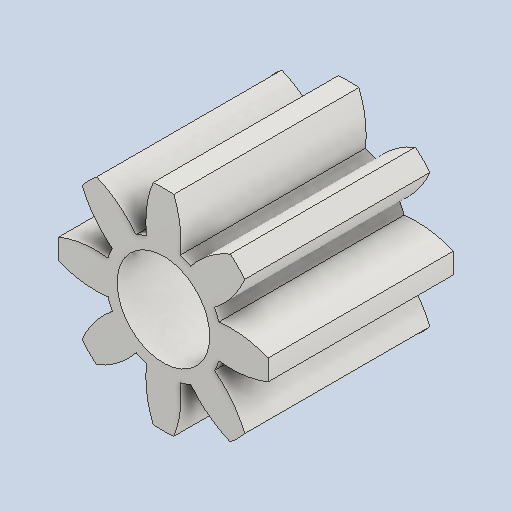
# Autodesk Inventor part: Spur Gear1
Saved by Autodesk Inventor 2022.3 (Build 263350000, 350)
## iProperties
CustomPartVersion: 1
Created: 2023-01-16
Part Number: Spur Gear1
Material: Steel
Document SubType Name: Modeling
Designer: komputer
Categories: <?xml version="1.0" encoding="UTF-16"?> <MemberInstance><Categories><FamilyTemplate><FamilyTemplateParameter ValueType="xs:double" Id="1" ObjectReferenceKey="da_z" ObjectType="kUserParameterObject"/><FamilyTemplateParameter ValueType="xs:double" Id="2" ObjectReferenceKey="da_b" ObjectType="kUserParameterObject"/><FamilyTemplateParameter ValueType="xs:double" Id="3" ObjectReferenceKey="da_beta" ObjectType="kUserParameterObject"/><FamilyTemplateParameter ValueType="xs:double" Id="4" ObjectReferenceKey="da_da" ObjectType="kUserParameterObject"/><FamilyTemplateParameter ValueType="xs:double" Id="5" ObjectReferenceKey="da_aw" ObjectType="kUserParameterObject"/><FamilyTemplateParameter ValueType="xs:string" Id="6" ObjectReferenceKey="EAIAABAAAACIAQAAAAAAAIAAAAAAAAAA" ObjectType="83910656" SubObjectId="SurfaceGeometry"/></FamilyTemplate><ParamToTemplateMap><ParamToTemplate CategoryParameter="//CategoryParameter[@InternalName='046C89C9-8512-4d59-83FE-43B91F4F132A']" TemplateParameter="1"/><ParamToTemplate CategoryParameter="//CategoryParameter[@InternalName='2552DF32-E462-4b46-AEBF-C6C7768E72AC']" TemplateParameter="2"/><ParamToTemplate CategoryParameter="//CategoryParameter[@InternalName='C9EE641D-15FC-4fae-A226-E94C4372FDD7']" TemplateParameter="3"/><ParamToTemplate><ParamToTemplate CategoryParameter="//CategoryParameter[@InternalName='00B6519A-459B-49c7-AD84-2E56D39A5744']" ConstantValue="0.000000"/></ParamToTemplate><ParamToTemplate><ParamToTemplate CategoryParameter="//CategoryParameter[@InternalName='04B31F0E-C7A6-4894-AA32-9629BEFACF47']" ConstantValue="1.000000"/></ParamToTemplate><ParamToTemplate><ParamToTemplate CategoryParameter="//CategoryParameter[@InternalName='43CBEC2E-7847-49e7-A936-2F7889FCB2D9']" ConstantValue="0.250000"/></ParamToTemplate><ParamToTemplate><ParamToTemplate CategoryParameter="//CategoryParameter[@InternalName='B1EFC894-105D-4ebd-86BF-FA20ED196853']" ConstantValue="0.350000"/></ParamToTemplate><ParamToTemplate><ParamToTemplate CategoryParameter="//CategoryParameter[@InternalName='51175063-3D10-4879-93E8-6246FE8B403D']" ConstantValue="2060000000.000000"/></ParamToTemplate><ParamToTemplate><ParamToTemplate CategoryParameter="//CategoryParameter[@InternalName='A3A52E27-4454-46a9-B0BD-C932399B70AF']" ConstantValue="0.300000"/></ParamToTemplate><ParamToTemplate><ParamToTemplate CategoryParameter="//CategoryParameter[@InternalName='91B76062-C214-41d9-B1B9-14D2AB99603D']" ConstantValue="0.045480"/></ParamToTemplate><ParamToTemplate><ParamToTemplate CategoryParameter="//CategoryParameter[@InternalName='374E806E-8B8A-4dda-A9AA-1039D6500AD2']" ConstantValue="21.987687"/></ParamToTemplate><ParamToTemplate><ParamToTemplate CategoryParameter="//CategoryParameter[@InternalName='2D373A89-B862-43d6-8D0B-0CBF12AB9F6C']" ConstantValue="0.349066"/></ParamToTemplate><ParamToTemplate CategoryParameter="//CategoryParameter[@InternalName='37777632-D6A2-4fac-9D53-DB8ACD95C989']" TemplateParameter="4"/><ParamToTemplate CategoryParameter="//CategoryParameter[@InternalName='FD1017F1-B727-4f7e-9707-0F86F1FF9423']" TemplateParameter="5"/><ParamToTemplate><ParamToTemplate CategoryParameter="//CategoryParameter[@InternalName='9E1B4470-B2D3-4ff1-B813-535BB4CDF51A']" ConstantValue="3520000.000000"/></ParamToTemplate><ParamToTemplate><ParamToTemplate CategoryParameter="//CategoryParameter[@InternalName='F8452263-BFF6-458c-9FB1-07C4B99E95CD']" ConstantValue="11400000.000000"/></ParamToTemplate><ParamToTemplate><ParamToTemplate CategoryParameter="//CategoryParameter[@InternalName='3E3BB259-FD49-497f-8171-6EBC954A3479']" ConstantValue="2.000000"/></ParamToTemplate><ParamToTemplate CategoryParameter="//CategoryParameter[@InternalName='27C3BAF2-7550-4e4b-AE2C-0DB134B7D9B7']" TemplateParameter="6"/></ParamToTemplateMap><Category DisplayName="Gear" InternalName="DC85795E-93AB-48d5-8EEE-5A27447B64BD" Mnemonic="Gear"><CategoryParameter DisplayName="z" InternalName="046C89C9-8512-4d59-83FE-43B91F4F132A" Mnemonic="z"/><CategoryParameter DisplayName="b" InternalName="2552DF32-E462-4b46-AEBF-C6C7768E72AC" Mnemonic="b"/><CategoryParameter DisplayName="||b|" InternalName="C9EE641D-15FC-4fae-A226-E94C4372FDD7" Mnemonic="beta"/><CategoryParameter DisplayName="x" InternalName="00B6519A-459B-49c7-AD84-2E56D39A5744" Mnemonic="x"/><CategoryParameter DisplayName="a*" InternalName="04B31F0E-C7A6-4894-AA32-9629BEFACF47" Mnemonic="a"/><CategoryParameter DisplayName="c*" InternalName="43CBEC2E-7847-49e7-A936-2F7889FCB2D9" Mnemonic="c"/><CategoryParameter DisplayName="r|.f|*" InternalName="B1EFC894-105D-4ebd-86BF-FA20ED196853" Mnemonic="rf"/><CategoryParameter DisplayName="E" InternalName="51175063-3D10-4879-93E8-6246FE8B403D" Mnemonic="E"/><CategoryParameter DisplayName="||m|" InternalName="A3A52E27-4454-46a9-B0BD-C932399B70AF" Mnemonic="mi"/><Category DisplayName="SpurGear" InternalName="26C5A22E-A91E-4dfd-A3B3-23CCAFAE1764" Mnemonic="SpurGear"><CategoryParameter DisplayName="m" InternalName="91B76062-C214-41d9-B1B9-14D2AB99603D" Mnemonic="m"/><CategoryParameter DisplayName="P" InternalName="374E806E-8B8A-4dda-A9AA-1039D6500AD2" Mnemonic="PP"/><CategoryParameter DisplayName="||a|" InternalName="2D373A89-B862-43d6-8D0B-0CBF12AB9F6C" Mnemonic="alpha"/><CategoryParameter DisplayName="d|.a|" InternalName="37777632-D6A2-4fac-9D53-DB8ACD95C989" Mnemonic="da"/><CategoryParameter DisplayName="a|.w|" InternalName="FD1017F1-B727-4f7e-9707-0F86F1FF9423" Mnemonic="aw"/><CategoryParameter DisplayName="||s||.Flim|" InternalName="9E1B4470-B2D3-4ff1-B813-535BB4CDF51A" Mnemonic="sFlim"/><CategoryParameter DisplayName="||s||.Hlim|" InternalName="F8452263-BFF6-458c-9FB1-07C4B99E95CD" Mnemonic="sHlim"/><CategoryParameter DisplayName="type" InternalName="3E3BB259-FD49-497f-8171-6EBC954A3479" Mnemonic="type"/><CategoryParameter DisplayName="PitchDiameter" InternalName="27C3BAF2-7550-4e4b-AE2C-0DB134B7D9B7" Mnemonic="IDS_PITCHDIAM"/></Category></Category></Categories></MemberInstance>
Density: 1 g/cm^3
Appearance: Steel
Author: komputer
Autodesk Inventor part; units mm, degrees
sketch "Sketch1" plane through (0, 0, 0) normal (0, 0, 1) x (1, 0, 0)
  circle A0 centre (0, 0) radius 2.274
  dimension "d0" = 4.548
  constraints: 1 centre point
  measures "d0" diameter of A0
extrude "Extrusion1" add sketch "Sketch1" along normal blind 20
ref_plane "Work Plane2" through (0, 0, 10) normal (0, 0, 1) x (1, 0, 0)
sketch "Sketch2" plane through (0, 0, 0) normal (0, 0, -1) x (-1, 0, 0)
  circle A0 centre (0, 0) radius 2.274 projected
  circle A1 centre (0, 0) radius 1.8192
  dimension "d3" = 3.6384
  constraints: 1 centre point, 1 coincident
  measures "d3" diameter of A1
surface extrude "Pitch Diameter" sketch "Sketch2" against normal through all shown no curves A1
ref_plane "Work Plane8" through (0, 0, 0) normal (0.9238795, 0.3826834, 0) x (0, 0, 1)
ref_plane "Work Plane9" through (0, 0, 0) normal (1, 0, 0) x (0, 1, 0)
spur gear teeth "Spur Gear" teeth 8 pitch diameter 3.6384 tip diameter 4.548 root diameter 2.5014 face width 20 start plane through (0, 0, 0) normal (0, 0, -1) x (-1, 0, 0)
sketch "Sketch3" plane through (0, 0, 20) normal (0, 0, 1) x (1, 0, 0)
  arc A0 (-1.7578, 1.4426) -> (-1.103, 0.5896) centre (0.2047, 2.2712) ccw projected
  arc A1 (-1.103, 0.5896) -> (-1.1968, 0.3631) centre (0, 0) ccw projected
  arc A2 (-1.1968, 0.3631) -> (-2.2631, 0.2229) centre (-1.4613, -1.7508) ccw projected
  arc A3 (-2.2631, 0.2229) -> (-2.2631, -0.2229) centre (0, 0) ccw projected
  arc A4 (-2.2631, -0.2229) -> (-1.1968, -0.3631) centre (-1.4613, 1.7508) ccw projected
  arc A5 (-1.1968, -0.3631) -> (-1.103, -0.5896) centre (0, 0) ccw projected
  arc A6 (-1.103, -0.5896) -> (-1.7578, -1.4426) centre (0.2047, -2.2712) ccw projected
  arc A7 (-1.7578, -1.4426) -> (-1.4426, -1.7578) centre (0, 0) ccw projected
  arc A8 (-1.4426, -1.7578) -> (-0.5896, -1.103) centre (-2.2712, 0.2047) ccw projected
  arc A9 (-0.5896, -1.103) -> (-0.3631, -1.1968) centre (0, 0) ccw projected
  arc A10 (-0.3631, -1.1968) -> (-0.2229, -2.2631) centre (1.7508, -1.4613) ccw projected
  arc A11 (-0.2229, -2.2631) -> (0.2229, -2.2631) centre (0, 0) ccw projected
  arc A12 (0.2229, -2.2631) -> (0.3631, -1.1968) centre (-1.7508, -1.4613) ccw projected
  arc A13 (0.3631, -1.1968) -> (0.5896, -1.103) centre (0, 0) ccw projected
  arc A14 (0.5896, -1.103) -> (1.4426, -1.7578) centre (2.2712, 0.2047) ccw projected
  arc A15 (1.4426, -1.7578) -> (1.7578, -1.4426) centre (0, 0) ccw projected
  arc A16 (1.7578, -1.4426) -> (1.103, -0.5896) centre (-0.2047, -2.2712) ccw projected
  arc A17 (1.103, -0.5896) -> (1.1968, -0.3631) centre (0, 0) ccw projected
  arc A18 (1.1968, -0.3631) -> (2.2631, -0.2229) centre (1.4613, 1.7508) ccw projected
  arc A19 (2.2631, -0.2229) -> (2.2631, 0.2229) centre (0, 0) ccw projected
  arc A20 (2.2631, 0.2229) -> (1.1968, 0.3631) centre (1.4613, -1.7508) ccw projected
  arc A21 (1.1968, 0.3631) -> (1.103, 0.5896) centre (0, 0) ccw projected
  arc A22 (1.103, 0.5896) -> (1.7578, 1.4426) centre (-0.2047, 2.2712) ccw projected
  arc A23 (1.7578, 1.4426) -> (1.4426, 1.7578) centre (0, 0) ccw projected
  arc A24 (1.4426, 1.7578) -> (0.5896, 1.103) centre (2.2712, -0.2047) ccw projected
  arc A25 (0.5896, 1.103) -> (0.3631, 1.1968) centre (0, 0) ccw projected
  arc A26 (0.3631, 1.1968) -> (0.2229, 2.2631) centre (-1.7508, 1.4613) ccw projected
  arc A27 (0.2229, 2.2631) -> (-0.2229, 2.2631) centre (0, 0) ccw projected
  arc A28 (-0.2229, 2.2631) -> (-0.3631, 1.1968) centre (1.7508, 1.4613) ccw projected
  arc A29 (-0.3631, 1.1968) -> (-0.5896, 1.103) centre (0, 0) ccw projected
  arc A30 (-0.5896, 1.103) -> (-1.4426, 1.7578) centre (-2.2712, -0.2047) ccw projected
  arc A31 (-1.4426, 1.7578) -> (-1.7578, 1.4426) centre (0, 0) ccw projected
ref_plane "Work Plane11" through (-4.2612, 0.6505, 4) normal (0, 0, 1) x (0.9749279, -0.2225209, 0)
extrude "Extrusion2" cut sketch "Sketch3" against normal up to surface (16 mm away)
sketch "Sketch4" plane through (0, 0, 4) normal (0, 0, 1) x (1, 0, 0)
  arc A0 (-1.1968, 0.3631) -> (-2.2631, 0.2229) centre (-1.4613, -1.7508) ccw projected
  arc A1 (-2.2631, 0.2229) -> (-2.2631, -0.2229) centre (0, 0) ccw projected
  arc A2 (-2.2631, -0.2229) -> (-1.1968, -0.3631) centre (-1.4613, 1.7508) ccw projected
  arc A3 (-1.1968, -0.3631) -> (-1.103, -0.5896) centre (0, 0) ccw projected
  arc A4 (-1.103, -0.5896) -> (-1.7578, -1.4426) centre (0.2047, -2.2712) ccw projected
  arc A5 (-1.7578, -1.4426) -> (-1.4426, -1.7578) centre (0, 0) ccw projected
  arc A6 (-1.4426, -1.7578) -> (-0.5896, -1.103) centre (-2.2712, 0.2047) ccw projected
  arc A7 (-0.5896, -1.103) -> (-0.3631, -1.1968) centre (0, 0) ccw projected
  arc A8 (-0.3631, -1.1968) -> (-0.2229, -2.2631) centre (1.7508, -1.4613) ccw projected
  arc A9 (-0.2229, -2.2631) -> (0.2229, -2.2631) centre (0, 0) ccw projected
  arc A10 (0.2229, -2.2631) -> (0.3631, -1.1968) centre (-1.7508, -1.4613) ccw projected
  arc A11 (0.3631, -1.1968) -> (0.5896, -1.103) centre (0, 0) ccw projected
  arc A12 (0.5896, -1.103) -> (1.4426, -1.7578) centre (2.2712, 0.2047) ccw projected
  arc A13 (1.4426, -1.7578) -> (1.7578, -1.4426) centre (0, 0) ccw projected
  arc A14 (1.7578, -1.4426) -> (1.103, -0.5896) centre (-0.2047, -2.2712) ccw projected
  arc A15 (1.103, -0.5896) -> (1.1968, -0.3631) centre (0, 0) ccw projected
  arc A16 (1.1968, -0.3631) -> (2.2631, -0.2229) centre (1.4613, 1.7508) ccw projected
  arc A17 (2.2631, -0.2229) -> (2.2631, 0.2229) centre (0, 0) ccw projected
  arc A18 (2.2631, 0.2229) -> (1.1968, 0.3631) centre (1.4613, -1.7508) ccw projected
  arc A19 (1.1968, 0.3631) -> (1.103, 0.5896) centre (0, 0) ccw projected
  arc A20 (1.103, 0.5896) -> (1.7578, 1.4426) centre (-0.2047, 2.2712) ccw projected
  arc A21 (1.7578, 1.4426) -> (1.4426, 1.7578) centre (0, 0) ccw projected
  arc A22 (1.4426, 1.7578) -> (0.5896, 1.103) centre (2.2712, -0.2047) ccw projected
  arc A23 (0.5896, 1.103) -> (0.3631, 1.1968) centre (0, 0) ccw projected
  arc A24 (0.3631, 1.1968) -> (0.2229, 2.2631) centre (-1.7508, 1.4613) ccw projected
  arc A25 (0.2229, 2.2631) -> (-0.2229, 2.2631) centre (0, 0) ccw projected
  arc A26 (-0.2229, 2.2631) -> (-0.3631, 1.1968) centre (1.7508, 1.4613) ccw projected
  arc A27 (-0.3631, 1.1968) -> (-0.5896, 1.103) centre (0, 0) ccw projected
  arc A28 (-0.5896, 1.103) -> (-1.4426, 1.7578) centre (-2.2712, -0.2047) ccw projected
  arc A29 (-1.4426, 1.7578) -> (-1.7578, 1.4426) centre (0, 0) ccw projected
  arc A30 (-1.7578, 1.4426) -> (-1.103, 0.5896) centre (0.2047, 2.2712) ccw projected
  arc A31 (-1.103, 0.5896) -> (-1.1968, 0.3631) centre (0, 0) ccw projected
  circle A32 centre (0, 0) radius 1
  dimension "d51" = 2
  constraints: 1 centre point, 1 coincident
  measures "d51" diameter of A32
extrude "Extrusion3" cut sketch "Sketch4" against normal through all contours A32
equation "\"d0\" = da_da"
equation "\"d1\" = da_b"
equation "\"d3\" = da_d"
equation "\"d16\" = da_aw"
equation "\"d43\" = da_aw"
equation "\"d46\" = da_aw"
equation "\"da_da\" = 4.548"
equation "\"da_b\" = 20"
equation "\"da_d\" = 3.6384"
equation "\"da_aw\" = 5.0028"
body "Solid1"
body "Srf1"
